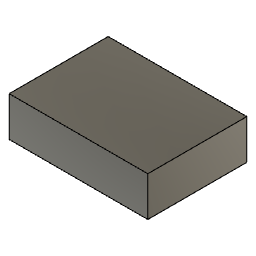
Pin Support v0 (Autodesk Fusion 360 design; units mm, degrees)
Autodesk Fusion 360 part; units mm, degrees
sketch "Sketch1" plane through (0, 0, 0) normal (0, 0, 1) x (1, 0, 0)
  line L0 (-25, 25) -> (-18, 25)
  line L1 (-18, 25) -> (-18, 20)
  line L2 (-18, 20) -> (-25, 20)
  line L3 (-25, 20) -> (-25, 25)
  circle A0 centre (-21.5, 22.5) radius 2
  dimension "d1" = 7
  dimension "d2" = 5
  dimension "d3" = 4
  constraint horizontal L0
  constraint vertical L1
  constraint horizontal L2
  constraint vertical L3
  measures "d1" distance of L0.start L0.end
  measures "d2" distance of L0.start L2.end
  measures "d3" diameter of A0
extrude "Extrude1" add sketch "Sketch1" along normal blind 2
sketch "Sketch2" plane through (0, 0, 2) normal (0, 0, 1) x (-1, 0, 0)
  circle A0 centre (21.5, -22.5) radius 2
  line L0 (25, -20) -> (18, -20)
  line L1 (18, -20) -> (18, -25)
  line L2 (18, -25) -> (25, -25)
  line L3 (25, -25) -> (25, -20)
  circle A1 centre (21.5, -22.5) radius 2
  constraint concentric A0 A1
extrude "Extrude2" add sketch "Sketch2" against normal blind 1 contours A0 A1
